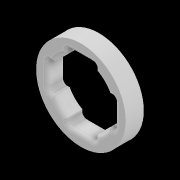
# Autodesk Inventor part: Distans_Axel_parametriserad_05 [2020-11-24]
Saved by Autodesk Inventor 2020 (Build 240168000, 168)
## iProperties
Created: 2020-11-24
Part Number: Distans_Axel_parametriserad_05 [2020-11-24]
Material: Generic
Document SubType Name: Modeling
Designer: Gottfrid
Density: 1 g/cm^3
Appearance: Default
Author: Gottfrid
Autodesk Inventor part; units mm, degrees
ref_plane "YZ Plane" through (0, 0, 0) normal (1, 0, 0) x (0, 1, 0)
ref_plane "XZ Plane" through (0, 0, 0) normal (0, 1, 0) x (-1, 0, 0)
ref_plane "XY Plane" through (0, 0, 0) normal (0, 0, 1) x (1, 0, 0)
sketch "Sketch1" plane through (0, 0, 0) normal (0, 0, 1) x (1, 0, 0)
  circle A0 centre (0, 0) radius 3.5
  circle A1 centre (0, 0) radius 5
  line L0 (-1.2333, -3.7857) -> (1.2333, -3.7857)
  line L1 (1.6333, -3.3857) -> (1.6333, 3.3857)
  line L2 (1.2333, 3.7857) -> (-1.2333, 3.7857)
  line L3 (-1.6333, 3.3857) -> (-1.6333, -3.3857)
  line L4 (-1.6333, -3.7857) -> (1.6333, 3.7857) construction
  line L5 (1.6333, -3.7857) -> (-1.6333, 3.7857) construction
  line L6 (-3.3857, 1.6333) -> (3.3857, 1.6333)
  line L7 (3.7857, 1.2333) -> (3.7857, -1.2333)
  line L8 (3.3857, -1.6333) -> (-3.3857, -1.6333)
  line L9 (-3.7857, -1.2333) -> (-3.7857, 1.2333)
  line L10 (-3.7857, 1.6333) -> (3.7857, -1.6333) construction
  line L11 (3.7857, 1.6333) -> (-3.7857, -1.6333) construction
  arc A2 (-1.2333, 3.7857) -> (-1.6333, 3.3857) centre (-1.2333, 3.3857) ccw
  arc A3 (1.6333, 3.3857) -> (1.2333, 3.7857) centre (1.2333, 3.3857) ccw
  arc A4 (1.2333, -3.7857) -> (1.6333, -3.3857) centre (1.2333, -3.3857) ccw
  arc A5 (-1.6333, -3.3857) -> (-1.2333, -3.7857) centre (-1.2333, -3.3857) ccw
  arc A6 (3.7857, 1.2333) -> (3.3857, 1.6333) centre (3.3857, 1.2333) ccw
  arc A7 (3.3857, -1.6333) -> (3.7857, -1.2333) centre (3.3857, -1.2333) ccw
  arc A8 (-3.7857, -1.2333) -> (-3.3857, -1.6333) centre (-3.3857, -1.2333) ccw
  arc A9 (-3.3857, 1.6333) -> (-3.7857, 1.2333) centre (-3.3857, 1.2333) ccw
  point P0 (-1.6333, -3.0955)
  point P1 (-3.0955, -1.6333)
  point P2 (-3.0955, 1.6333)
  point P3 (-1.6333, 3.0955)
  point P4 (1.6333, 3.0955)
  point P5 (3.0955, 1.6333)
  point P6 (3.0955, -1.6333)
  point P7 (1.6333, -3.0955)
  dimension "d0" = 10
  dimension "d1" = 7
  dimension "d2" = 7.5714
  dimension "d3" = 7.5714
  dimension "d4" = 3.2667
  dimension "d5" = 3.2667
  dimension "d6" = 0.4
  constraints: 24 end point, 16 point on circle, 16 point on line, 16 tangent, 10 centre point, 7 equal radius, 4 midpoint, 4 parallel, 2 coincident, 2 horizontal, 2 perpendicular
  measures "d0" diameter of A1
  measures "d1" diameter of A0
  measures "d2" distance between parallel lines of L0 L2
  measures "d3" distance between parallel lines of L9 L7
  measures "d4" distance between parallel lines of L1 L3
  measures "d5" distance between parallel lines of L8 L6
  measures "d6" radius of A2
extrude "Extrusion1" add sketch "Sketch1" along normal blind 2
fillet "Fillet1" radius 0.4 48 edges at (1.5162, 3.6686, 2) (1.6333, 3.2406, 2) (-1.5162, 3.6686, 2) (-1.6333, 3.2406, 2) (0, 3.7857, 2) (-3.6686, 1.5162, 2) (-3.2406, 1.6333, 2) (-3.6686, -1.5162, 2) (-3.2406, -1.6333, 2) (-3.7857, 0, 2) (-1.5162, -3.6686, 2) (-1.6333, -3.2406, 2) (1.5162, -3.6686, 2) (1.6333, -3.2406, 2) (0, -3.7857, 2) (3.6686, -1.5162, 2) (3.2406, -1.6333, 2) (3.6686, 1.5162, 2) (3.2406, 1.6333, 2) (3.7857, 0, 2) (-2.4749, 2.4749, 2) (2.4749, 2.4749, 2) (2.4749, -2.4749, 2) (-2.4749, -2.4749, 2) (-2.4749, 2.4749, 0) (1.5162, 3.6686, 0) (1.6333, 3.2406, 0) (-1.5162, 3.6686, 0) (-1.6333, 3.2406, 0) (0, 3.7857, 0) (2.4749, 2.4749, 0) (2.4749, -2.4749, 0) (3.6686, -1.5162, 0) (3.2406, -1.6333, 0) (3.6686, 1.5162, 0) (3.2406, 1.6333, 0) (3.7857, 0, 0) (-1.5162, -3.6686, 0) (-1.6333, -3.2406, 0) (1.5162, -3.6686, 0) (1.6333, -3.2406, 0) (0, -3.7857, 0) (-2.4749, -2.4749, 0) (-3.6686, 1.5162, 0) (-3.2406, 1.6333, 0) (-3.6686, -1.5162, 0) (-3.2406, -1.6333, 0) (-3.7857, 0, 0)
equation "\"d0\" = D_axel + d_axelRing"
equation "\"d1\" = D_axel"
equation "\"d6\" = r_filletAxel"
equation "\"d7\" = h_distansAxel"
equation "\"d9\" = r_filletDistansAxel"
equation "\"h_distansAxel\" = 2"
equation "\"r_filletDistansAxel\" = 0.4"
equation "\"D_axel\" = 7"
equation "\"d_axelRing\" = 3"
equation "\"r_filletAxel\" = 0.4"
body "Solid1"
